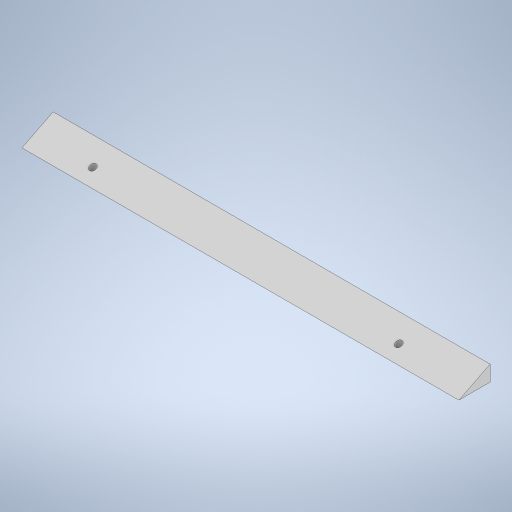
# Autodesk Inventor part: paw shelf_v01
Saved by Autodesk Inventor 2023 (Build 270158000, 158)
## iProperties
Created: 2023-02-22
Part Number: paw shelf_v01
Material: Generic
Document SubType Name: Modeling
Designer: Akramilab
Density: 1 g/cm^3
Appearance: Default
Author: Akramilab
Autodesk Inventor part; units mm, degrees
ref_plane "YZ Plane" through (0, 0, 0) normal (1, 0, 0) x (0, 1, 0)
ref_plane "XZ Plane" through (0, 0, 0) normal (0, 1, 0) x (-1, 0, 0)
ref_plane "XY Plane" through (0, 0, 0) normal (0, 0, 1) x (1, 0, 0)
sketch "Sketch1" plane through (0, 0, 0) normal (0, 0, 1) x (1, 0, 0)
  line L0 (140, 5) -> (-140, 5)
  line L1 (-140, 5) -> (-140, -5)
  line L2 (-140, -5) -> (140, -5)
  line L3 (140, -5) -> (140, 5)
  line L4 (140, 5) -> (-140, -5) construction
  line L5 (-140, 5) -> (140, -5) construction
  point P0 (0, 0)
  dimension "d0" = 280
  dimension "d1" = 10
  constraints: 12 end point, 2 midpoint, 2 parallel, 1 horizontal, 1 perpendicular
  measures "d0" distance of L2.end L1.end
  measures "d1" distance of L1.end L0.end
extrude "Extrusion1" add sketch "Sketch1" along normal blind 20
sketch "Sketch3" plane through (-140, -5, 0) normal (-1, 0, 0) x (0, 0, 1)
  line L0 (0, 10) -> (0, 0) projected
  line L1 (20, 10) -> (20, 0) projected
  line L2 (0, 10) -> (20, 0)
  line L3 (20, 0) -> (20, 10)
  line L4 (0, 10) -> (20, 10) projected
  line L5 (20, 10) -> (0, 10)
  point P0 (0, 5)
  constraints: 6 end point, 1 collinear, 1 perpendicular
extrude "Extrusion3" cut sketch "Sketch3" against normal through all
sketch "Sketch5" plane through (-140, -5, 0) normal (0, -1, 0) x (1, 0, 0)
  circle A0 centre (37.5, 12) radius 2
  circle A1 centre (233.5, 12) radius 2
  line L0 (0, 20) -> (280, 20) projected
  line L1 (0, 0) -> (0, 20) projected
  point P0 (140, 0)
  dimension "d8" = 4
  dimension "d9" = 4
  dimension "d10" = 196
  dimension "d11" = 8
  dimension "d12" = 8
  dimension "d13" = 37.5
  constraints: 2 centre point
  measures "d8" diameter of A0
  measures "d9" diameter of A1
  measures "d10" distance of A1.centre A0.centre
  measures "d11" distance from line of L0 A0.centre
  measures "d12" distance from line of L0 A1.centre
  measures "d13" distance from line of L1 A0.centre
hole "Hole1" at (93.5, -5, 12) at (-102.5, -5, 12) direction (0, 1, 0) diameter 4 depth 5 tip angle 118
body "Solid1"
